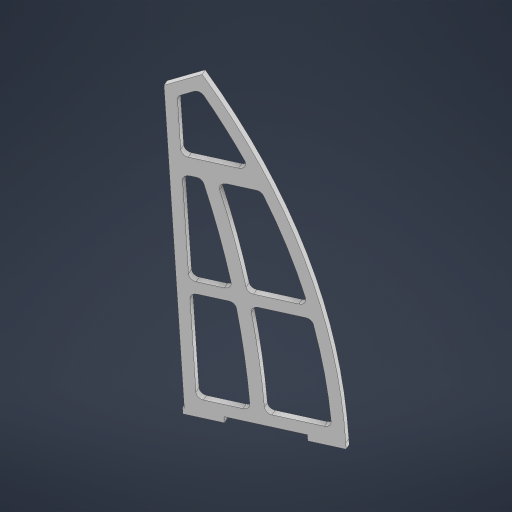
# Autodesk Inventor part: sponson_spanner_bottom
Saved by Autodesk Inventor 2023 (Build 270158030, 158C)
## iProperties
Created: 2022-03-22
Part Number: sponson_spanner_bottom
Material: Generic
Document SubType Name: Modeling
Designer: kardo
Density: 1 g/cm^3
Appearance: Default
Mass: 2.79206 g
Surface Area: 40.129 cm^2
Volume: 2.79206 cm^3
Author: kardo
Autodesk Inventor part; units mm, degrees
ref_plane "YZ Plane" through (0, 0, 0) normal (1, 0, 0) x (0, 1, 0)
ref_plane "XZ Plane" through (0, 0, 0) normal (0, 1, 0) x (-1, 0, 0)
ref_plane "XY Plane" through (0, 0, 0) normal (0, 0, 1) x (1, 0, 0)
derived "parameters_frame.ipt"
derived "stencil_frame.ipt"
sketch "sk_joint_locations" plane through (81.12, 0, 0) normal (1, 0, 0) x (0, 1, 0)
  line L0 (0, 0) -> (122.4, 8.559) construction
  line L1 (36.465, 28.832) -> (112.2, 28.832) construction
  arc A0 (36.465, 28.832) -> (11.22, 28.376) centre (36.465, -670.197) ccw construction
  line L2 (-241.5001, 19.2432) -> (11.22, 28.376) construction
  line L3 (-345, 16.32) -> (-262.2001, 18.586) construction
  arc A1 (-262.2001, 18.586) -> (-241.5001, 19.2432) centre (-326.8578, 2381.2399) ccw construction
  line L4 (-95.1358, 3119.4657) -> (254.2444, -1876.9042) construction
  line L5 (-230.0001, 3089.1136) -> (-230.0001, -1866.0023) construction
  line L6 (-114.9999, 3089.1136) -> (-114.9999, -1866.0023) construction
  line L7 (-345, 3089.1136) -> (-345, -1866.0023) construction
  line L8 (0, 3089.1136) -> (0, -1866.0023) construction
  line L9 (516.4305, 45.5774) -> (-594.5903, 6.7797) construction
  line L10 (-657.7604, -27.3784) -> (621.8174, 62.0984) construction
  line L11 (193.4506, 30.2962) -> (193.1714, 38.2913) construction
  line L12 (201.1621, 36.7028) -> (201.7215, 28.7028) construction
  line L13 (0, 14.96) -> (121.9304, 15.2746) construction
  line L14 (-230.0001, 45.8702) -> (-230.0001, 19.6588) construction
  line L15 (-345, 37.4554) -> (-345, 16.32) construction
  line L16 (-114.9999, 51.0173) -> (-114.9999, 23.8147) construction
  line L17 (0, 52.89) -> (0, 27.9705) construction
  line L18 (119.462, 50.575) -> (119.9556, 43.5149) construction
  line L19 (120.4493, 36.4549) -> (119.9556, 43.5149) construction
  line L20 (120.4493, 36.4549) -> (120.943, 29.3948) construction
  line L21 (120.943, 29.3948) -> (121.4367, 22.3347) construction
  line L22 (121.4367, 22.3347) -> (121.9304, 15.2746) construction
  line L23 (0, 14.96) -> (0, 0) construction
  line L24 (112.2, 37.536) -> (112.2, 28.832) construction
  line L25 (112.2, 35.548) -> (112.2, 30.82) construction
  spline S0 degree 4 poles (-345, 37.4554) (-258.8682, 45.1562) (-172.5926, 49.7838) (-86.3161, 52.89) (0, 52.89) knots 0 0 0 0 0 1 1 1 1 1
  spline S1 degree 3 poles (0, 52.89) (92.8353, 52.89) (195.0311, 49.5089) (255, 36.448) knots 0 0 0 0 1 1 1 1
  spline S2 degree 2 poles (122.4, 8.559) (190.3044, 13.3074) (255, 36.448) knots 0 0 0 1 1 1
  point P0 (-95.1358, 3119.4657)
  point P1 (254.2444, -1876.9042)
  point P2 (193.311, 34.2938)
  point P3 (201.4418, 32.7028)
  point P4 (134.9575, 11.3411)
  point P5 (-345, 26.8877)
  point P6 (-230.0001, 32.7645)
  point P7 (-114.9999, 37.416)
  point P8 (0, 40.4303)
  point P9 (112.2, 33.184)
sketch "sk_spanner_joints_locations" plane through (0, 122.4, 8.559) normal (0, 0.9975641, 0.0697565) x (-1, 0, 0)
  line L0 (300.9234, 5.5808) -> (-420.7494, 38.9736) construction
  line L1 (-923.3057, -329.5522) -> (1264.6454, 574.8532) construction
  line L2 (-84.7099, 23.4246) -> (-83.6779, 17.514) construction
  line L3 (-84.7099, 23.4246) -> (-70.9223, 22.7866) construction
  line L4 (-83.6779, 17.514) -> (-70.9223, 22.7866) construction
  point P0 (0, 0)
  point P1 (-126.048, 0)
  point P2 (-156, 26.7233)
  point P3 (-141.742, 26.0635)
  point P4 (-98.9679, 24.0843)
  point P5 (-94.2704, 13.1355)
  point P6 (-115.4555, 4.3785)
ref_plane "plane_strnger_outer" through (84.12, 0, 0) normal (1, 0, 0) x (0, 1, 0)
sketch "sk_corner_offset" plane through (0, 122.4, 8.559) normal (0, 0.9975641, 0.0697565) x (-1, 0, 0)
  line L0 (-156, 26.7233) -> (-126.048, 0) construction
  line L1 (-126.048, 0) -> (-81.12, 0) construction
  point P0 (0, 0)
  point P1 (-125.5905, 1.2)
  dimension "d7" = 1.2
  dimension "d8" = 1.2
  constraints: 4 end point, 1 horizontal
  measures "d7" distance from line of L0 point (-125.59, 1.2)
  measures "d8" distance from line of point (-125.59, 1.2) L1
sketch "sk_tip_offset" plane through (81.12, 0, 0) normal (1, 0, 0) x (0, 1, 0)
  spline S0 degree 3 poles (0, 52.89) (92.8353, 52.89) (195.0311, 49.5089) (255, 36.448) knots 0 0 0 0 1 1 1 1 construction
  spline S1 degree 2 poles (122.4, 8.559) (190.3044, 13.3074) (255, 36.448) knots 0 0 0 1 1 1 construction
  spline S2 degree 5 poles (0, 51.69) (14.1108, 51.69) (28.2217, 51.6249) (42.3321, 51.4877) (70.2924, 51.0558) (98.2445, 50.2552) (112.0882, 49.7555) (138.5614, 48.5709) (165.0044, 46.8436) (177.6143, 45.8726) (199.84, 43.8477) (221.9828, 41.066) (231.553, 39.6839) (241.0942, 38.0879) (250.5671, 36.1558) knots 0 0 0 0 0 0 0.280662 0.280662 0.280662 0.556179 0.556179 0.556179 0.807705 0.807705 0.807705 1 1 1 1 1 1
  spline S3 degree 5 poles (122.3163, 9.7561) (148.5177, 11.5885) (174.5986, 15.1479) (200.4027, 20.4751) (225.7629, 27.5171) (250.5671, 36.1559) knots 0 0 0 0 0 0 1 1 1 1 1 1
  point P0 (0, 0)
  dimension "d9" = 1.2
  dimension "d10" = 1.2
  constraints: 1 coincident, 6 other
sketch "sk_spanner_bottom_base" plane through (126.048, 0, 0) normal (0.3820078, -0.0644661, 0.9219079) x (-0.1718217, 0.9752166, 0.139391)
  spline S0 degree 2 poles (120.5596, -22.8124) (192.7887, -36.4798) (261.4804, 0) knots 0 0 0 1 1 1 construction
  line L0 (-543.4693, 149.0099) -> (606.3971, -68.5694) projected
  line L1 (120.7234, -21.9466) -> (118.7583, -21.5747)
  line L2 (118.7583, -21.5747) -> (120.7254, -11.1786)
  line L3 (120.7254, -11.1786) -> (122.6906, -11.5505)
  line L4 (122.6906, -11.5505) -> (126.9526, 10.9734)
  line L5 (126.9526, 10.9734) -> (124.9875, 11.3453)
  line L6 (124.9875, 11.3453) -> (127.1185, 22.6072)
  line L7 (127.1185, 22.6072) -> (129.0836, 22.2354)
  line L8 (129.0836, 22.2354) -> (128.9946, 21.7653)
  line L9 (120.5596, -22.8124) -> (0, 0) construction
  spline S1 degree 2 poles (120.7234, -21.9466) (190.7476, -35.1967) (257.1166, 0.8326) knots 0 0 0 1 1 1
  point P0 (21.6578, 114.4574)
  point P1 (120.5596, -22.8124)
  point P2 (208.7275, 9.982)
  point P3 (256.8103, -2.4201)
  point P4 (0, 0)
  point P5 (252.5102, -1.6064)
  dimension "d4" = 2
  constraints: 16 end point, 3 parallel, 2 collinear, 2 perpendicular, 1 point on line, 5 other
  measures "d4" distance between parallel lines of L6 L4
extrude "thicken" add sketch "sk_spanner_bottom_base" along normal blind 2
sketch "sk_cut_weight" plane through (126.048, 0, 0) normal (0.3820078, -0.0644661, 0.9219079) x (-0.1718217, 0.9752166, 0.139391)
  spline S0 degree 2 poles (120.7234, -21.9466) (190.7476, -35.1967) (257.1166, 0.8326) knots 0 0 0 1 1 1 construction
  line L0 (-543.4693, 149.0099) -> (606.3971, -68.5694) projected
  line L1 (122.6906, -11.5505) -> (126.9526, 10.9734) construction
  line L2 (129.0836, 22.2354) -> (128.9946, 21.7653) projected
  line L3 (208.7275, 9.982) -> (203.0151, -20.207) construction
  line L4 (129.0836, 22.2354) -> (204.2826, 8.0061)
  line L5 (204.2826, 8.0061) -> (204.1937, 7.5361)
  line L6 (210.0891, 6.4205) -> (210.178, 6.8906)
  line L7 (210.178, 6.8906) -> (252.5991, -1.1364)
  line L8 (132.2702, 17.5615) -> (203.539, 4.0759)
  line L9 (203.539, 4.0759) -> (202.5191, -1.314)
  line L10 (132.2702, 17.5615) -> (129.5002, 2.9228)
  line L11 (209.4343, 2.9603) -> (205.8887, -15.7775)
  line L12 (252.5991, -1.1364) -> (252.5102, -1.6064)
  spline S1 degree 2 poles (124.8216, -0.2885) (164.8724, -7.867) (205.8713, -5.1125) knots 0 0 0 1 1 1
  line L13 (209.4343, 2.9603) -> (241.2974, -3.0688)
  line L14 (201.7529, -5.3633) -> (199.4904, -17.3202)
  line L15 (128.7565, -1.0077) -> (125.3312, -19.1097)
  line L16 (169.8697, 10.4468) -> (167.6246, -1.4181)
  line L17 (165.9394, 11.1905) -> (163.5983, -1.1818)
  line L18 (166.8742, -5.3839) -> (163.7642, -21.8193)
  line L19 (162.8491, -5.1411) -> (159.6785, -21.8971)
  line L20 (167.9046, 10.8187) -> (161.7193, -21.8693) construction
  line L21 (231.3886, 2.8771) -> (245.6475, -37.8741)
  line L22 (228.3757, -0.6238) -> (230.8093, -7.5787)
  line L23 (252.5991, -1.1364) -> (245.6475, -37.8741)
  spline S2 degree 5 poles (125.3312, -19.1096) (137.9928, -21.2536) (150.8208, -22.4121) (163.7291, -22.4855) (187.515, -20.5417) (210.6909, -14.9427) (221.1508, -11.626) (231.3603, -7.6431) (241.2974, -3.0688) knots 0 0 0 0 0 0 0.539997 0.539997 0.539997 1 1 1 1 1 1
  spline S3 degree 4 poles (125.5653, 3.6417) (134.9881, 1.8587) (144.4837, 0.4548) (154.0283, -0.5586) (163.5983, -1.1818) knots 0 0 0 0 0 1 1 1 1 1
  spline S4 degree 4 poles (163.5983, -1.1818) (173.314, -1.8146) (183.0558, -2.0452) (192.799, -1.8742) (202.5191, -1.314) knots 0 0 0 0 0 1 1 1 1 1
  point P0 (21.6578, 114.4574)
  point P1 (167.6246, -1.4181)
  point P2 (128.7343, 3.0587)
  point P3 (139.2857, 19.818)
  dimension "d11" = 3.6057
  dimension "d17" = 4
  dimension "d12" = 2
  dimension "d13" = 4
  dimension "d14" = 4
  dimension "d18" = 4
  dimension "d22" = 60
  dimension "d23" = 4
  dimension "d24" = 4
  constraints: 43 end point, 9 collinear, 7 point on line, 6 parallel, 5 perpendicular, 4 midpoint, 29 other
  measures "d12" distance between parallel lines of L6 L3
  measures "d13" distance between parallel lines of L3 L5
  measures "d14" distance between parallel lines of L4 L8
  measures "d18" distance between parallel lines of L17 L16
  measures "d22" angle of L7 L21
  measures "d23" distance between parallel lines of L22 L21
  measures "d24" distance between parallel lines of L1 L10
extrude "cut_weight" cut sketch "sk_cut_weight" along normal through all both and the other way through all contours L21 L7 L12 L0 | L0 L23 L21 S2 L13 | L13 S2 L21 | L22 S2 L11 L13 | L8 L17 S3 L10 | L8 L9 S4 L16 | S1 L19 S2 L15 | S1 L14 S2 L18
fillet "rounding" radius 2 20 edges at (87.7565, 203.5528, 31.1852) (87.7565, 163.3842, 28.3764) (102.6462, 163.8135, 22.2366) (105.2219, 125.7143, 18.5051) (87.7565, 125.2107, 25.707) (87.7565, 159.3939, 28.0973) (103.1174, 159.8368, 21.7633) (87.7565, 197.5674, 30.7667) (96.6346, 197.8234, 27.1058) (92.826, 197.7136, 28.6763) (107.8808, 198.1477, 22.4684) (118.8773, 160.2913, 15.2647) (99.3934, 159.7295, 23.2988) (105.3805, 204.061, 23.9179) (118.1047, 164.2592, 15.8623) (122.2479, 126.2052, 11.4845) (98.9161, 163.706, 23.7747) (101.525, 125.6077, 20.0296) (87.7565, 222.7834, 32.5299) (93.6537, 226.6286, 30.3552)
equation "\"d7\" = shell_thickness"
equation "\"d8\" = shell_thickness"
equation "\"d9\" = shell_thickness"
equation "\"d10\" = shell_thickness"
equation "\"d4\" = bulkhead_thickness"
equation "\"d5\" = bulkhead_thickness"
equation "\"d17\" = bulkhead_inset"
equation "\"d12\" = bulkhead_thickness"
equation "\"d13\" = 2 * bulkhead_thickness"
equation "\"d14\" = bulkhead_inset"
equation "\"d18\" = bulkhead_inset"
equation "\"d23\" = bulkhead_inset"
equation "\"d21\" = 0.5 * bulkhead_inset"
equation "\"d3\" = stringer_thickness"
equation "\"shell_thickness\" = 1.2"
equation "\"bulkhead_thickness\" = 2"
equation "\"bulkhead_inset\" = 4"
equation "\"stringer_thickness\" = 3"
body "Solid1"
